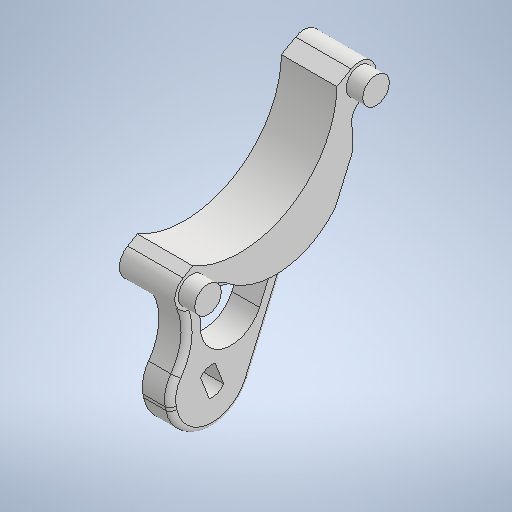
# Autodesk Inventor part: Jig
Saved by Autodesk Inventor 2025.2 (Build 292293000, 293)
## iProperties
Created: 2026-02-21
Part Number: Jig
Material: 一般
Document SubType Name: Modeling
Designer: naka6
Density: 1 g/cm^3
Appearance: 既定
Author: naka6
Autodesk Inventor part; units mm, degrees
ref_plane "YZ Plane" through (0, 0, 0) normal (1, 0, 0) x (0, 1, 0)
ref_plane "XZ Plane" through (0, 0, 0) normal (0, 1, 0) x (-1, 0, 0)
ref_plane "XY Plane" through (0, 0, 0) normal (0, 0, 1) x (1, 0, 0)
sketch "スケッチ1" plane through (0, 0, 0) normal (1, 0, 0) x (0, 1, 0)
  circle A0 centre (0, 0) radius 7.5
  circle A1 centre (0, 0) radius 2.6
  line L0 (0, 0) -> (40, 0)
  line L1 (21.0937, 8.7466) -> (38.5937, -21.5643)
  circle A2 centre (40, 0) radius 17.5
  circle A3 centre (21.0937, 8.7466) radius 3
  circle A4 centre (38.5937, -21.5643) radius 3
  line L2 (23.6918, 10.2466) -> (41.1918, -20.0643)
  line L3 (20.5133, 11.6899) -> (-1.4511, 7.3583)
  line L4 (37.4046, -24.3185) -> (-2.9729, -6.8856)
  line L5 (40, 0) -> (29.6077, -6)
  circle A5 centre (9.5821, 14.4722) radius 9.8569
  point P0 (39.7099, -17.4976)
  point P1 (24.7016, 8.4976)
  point P2 (33.2577, -13.3993)
  point P3 (37.2586, -14.7474)
  point P4 (18.9414, 11.3799)
  point P5 (2.0976, 8.0581)
  point P6 (18.4076, 10.0826)
  dimension "d0" = 15
  dimension "d1" = 5.2
  dimension "d2" = 40
  dimension "d3" = 35
  dimension "d5" = 35
  dimension "d6" = 6
  dimension "d7" = 6
  dimension "d14" = 120
  dimension "d15" = 12
  constraints: 12 end point, 8 tangent, 6 centre point, 6 point on circle, 5 coincident, 3 point on line, 1 horizontal, 1 perpendicular
  measures "d0" diameter of A0
  measures "d1" diameter of A1
  measures "d2" distance of L0.start L0.end
  measures "d3" distance of L1.start L1.end
  measures "d5" diameter of A2
  measures "d6" diameter of A3
  measures "d7" diameter of A4
  measures "d14" angle of L1 L0
  measures "d15" distance of L5.start L5.end
extrude "押し出し1" add sketch "スケッチ1" along normal blind 5 contours A0 | L3 A5 A0 | A0 L0 A2 L1 A4 L4 | A5 A3 L1 A2 L0 A0 | A4 | A3 | L1 A2 L2 A4 | A3 L2 A2 L1
sketch "スケッチ2" plane through (5, 0, 0) normal (1, 0, 0) x (0, 0, -1)
  arc A0 (24.3185, 37.4046) -> (20.0643, 41.1918) centre (21.5643, 38.5937) ccw projected
  line L0 (20.0643, 41.1918) -> (17.4976, 39.7099) projected
  arc A1 (-8.4976, 24.7016) -> (17.4976, 39.7099) centre (0, 40) ccw projected
  arc A2 (-10.2466, 23.6918) -> (-10.0826, 18.4076) centre (-8.7466, 21.0937) ccw projected
  line L1 (-8.0581, 2.0976) -> (-7.3583, -1.4511) projected
  arc A3 (-7.3583, -1.4511) -> (6.8856, -2.9729) centre (0, 0) ccw projected
  line L2 (6.8856, -2.9729) -> (24.3185, 37.4046) projected
  circle A4 centre (0, 0) radius 2.6 projected
  circle A5 centre (-8.7466, 21.0937) radius 3
  circle A6 centre (21.5643, 38.5937) radius 3
  line L3 (-8.4976, 24.7016) -> (-10.2466, 23.6918) projected
  arc A7 (-8.0581, 2.0976) -> (-10.0826, 18.4076) centre (-14.4722, 9.5821) ccw projected
  circle A8 centre (6.4088, 29.8437) radius 14
  circle A9 centre (-4.5271, 16.8281) radius 3
  circle A10 centre (23.1486, 32.8067) radius 3
  point P0 (-10.0826, 18.4076)
  point P1 (-6.6369, 18.9609)
  point P2 (-2.5972, 19.125)
  point P3 (17.207, 20.9331)
  point P4 (20.2992, 28.0951)
  point P5 (20.1945, 32.2838)
  point P6 (22.3564, 35.7002)
  dimension "d10" = 6
  dimension "d11" = 6
  dimension "d16" = 6
  dimension "d17" = 6
  dimension "d22" = 3
  dimension "d23" = 17.5
  dimension "d24" = 28
  constraints: 5 centre point, 4 tangent, 2 coincident
  measures "d10" diameter of A5
  measures "d11" diameter of A6
  measures "d16" diameter of A9
  measures "d17" diameter of A10
  measures "d22" distance from line of L0 A8.centre
  measures "d23" distance of A6.centre A8.centre
  measures "d24" diameter of A8
extrude "押し出し2" add sketch "スケッチ2" along normal blind 5 contours A6 A0 | A10 A8 A1 L0 A6 | A8 L2 A1 | A8 A9 A5 L3 A1 | A5 A2
sketch "スケッチ3" plane through (10, 0, 0) normal (1, 0, 0) x (0, 0, -1)
  arc A0 (22.3564, 35.7002) -> (20.0643, 41.1918) centre (21.5643, 38.5937) ccw projected
  circle A1 centre (21.5643, 38.5937) radius 2.4
  arc A2 (-10.2466, 23.6918) -> (-6.6369, 18.9609) centre (-8.7466, 21.0937) ccw projected
  circle A3 centre (-8.7466, 21.0937) radius 2.4
  point P0 (0, 0)
  dimension "d18" = 4.8
  dimension "d19" = 4.8
  constraints: 2 centre point, 2 coincident
  measures "d18" diameter of A1
  measures "d19" diameter of A3
extrude "押し出し3" add sketch "スケッチ3" along normal blind 3
sketch "スケッチ4" plane through (5, 0, 0) normal (1, 0, 0) x (0, 0, -1)
  circle A0 centre (0, 0) radius 2.6 projected
  line L0 (2.1005, -1.5322) -> (0.508, 2.5499)
  line L1 (-0.508, -2.5499) -> (-2.1005, 1.5322)
  line L2 (0.4478, 2.154) -> (1.7881, -1.2817) projected
  arc A1 (-0.4478, -2.154) -> (1.7881, -1.2817) centre (0, 0) ccw projected
  line L3 (-0.4478, -2.154) -> (-1.7881, 1.2817) projected
  arc A2 (0.4478, 2.154) -> (-1.7881, 1.2817) centre (0, 0) ccw projected
  dimension "d27" = 0.2
  dimension "d28" = 0.2
  constraints: 4 end point, 4 point on circle
  measures "d27" distance between parallel lines of L2 L0
  measures "d28" distance between parallel lines of L1 L3
extrude "押し出し4" add sketch "スケッチ4" against normal up to surface (5 mm away) contours A0 L0 | L1 A0
fillet "フィレット1" radius 6 1 edges at (2.5, 2.0976, 8.0581)
sketch "スケッチ5" plane through (5, 0, 0) normal (1, 0, 0) x (0, 0, -1)
  arc A0 (0.508, 2.5499) -> (-2.1005, 1.5322) centre (0, 0) ccw projected
  line L0 (0.508, 2.5499) -> (2.1005, -1.5322) projected
  arc A1 (-0.508, -2.5499) -> (2.1005, -1.5322) centre (0, 0) ccw projected
  line L1 (-0.508, -2.5499) -> (-2.1005, 1.5322) projected
  arc A2 (-6.4669, 3.8311) -> (-7.4807, -0.8305) centre (-1.5941, 0.3304) ccw projected
  line L2 (-7.4807, -0.8305) -> (-7.3583, -1.4511) projected
  arc A3 (-7.3583, -1.4511) -> (6.8856, -2.9729) centre (0, 0) ccw projected
  line L3 (6.8856, -2.9729) -> (17.207, 20.9331) projected
  arc A4 (-2.5972, 19.125) -> (17.207, 20.9331) centre (6.4088, 29.8437) ccw projected
  arc A5 (-2.5972, 19.125) -> (-6.6369, 18.9609) centre (-4.5271, 16.8281) ccw projected
  arc A6 (-10.0826, 18.4076) -> (-6.6369, 18.9609) centre (-8.7466, 21.0937) ccw projected
  arc A7 (-6.4669, 3.8311) -> (-10.0826, 18.4076) centre (-14.4722, 9.5821) ccw projected
  arc A8 (20.2992, 28.0951) -> (20.1945, 32.2838) centre (6.4088, 29.8437) ccw projected
  line L4 (20.2992, 28.0951) -> (24.3185, 37.4046) projected
  arc A9 (22.3564, 35.7002) -> (24.3185, 37.4046) centre (21.5643, 38.5937) ccw projected
  arc A10 (22.3564, 35.7002) -> (20.1945, 32.2838) centre (23.1486, 32.8067) ccw projected
  arc A11 (-4.2054, 17.2109) -> (-4.7866, 17.2555) centre (-4.5271, 16.8281) ccw
  arc A12 (-4.2054, 17.2109) -> (11.5638, 14.1697) centre (6.4088, 29.8437) ccw
  line L5 (11.5638, 14.1697) -> (4.5904, -1.9819)
  arc A13 (-4.9055, -0.9674) -> (4.5904, -1.9819) centre (0, 0) ccw
  line L6 (-4.9055, -0.9674) -> (-5.0279, -0.3468)
  arc A14 (-4.4366, 2.3725) -> (-5.0279, -0.3468) centre (-1.5941, 0.3304) ccw
  arc A15 (-4.4366, 2.3725) -> (-4.7866, 17.2555) centre (-14.4722, 9.5821) ccw
  circle A16 centre (3.4435, 9.3884) radius 5.5599
  circle A17 centre (-3.2484, 15.8531) radius 0.5
  circle A18 centre (10.6825, 13.3897) radius 0.5
  point P0 (-2.9643, 16.2645)
  point P1 (-3.6849, 15.6092)
  point P2 (-2.116, 9.4485)
  point P3 (8.548, 7.1845)
  point P4 (11.1415, 13.1915)
  point P5 (10.5568, 13.8736)
  dimension "d32" = 2.5
  dimension "d33" = 10
  dimension "d34" = 1
  dimension "d35" = 1
  constraints: 10 point on circle, 8 centre point, 6 tangent, 4 end point, 6 other
  measures "d32" radial gap between concentric circles of A7 A15
  measures "d33" distance of A16.centre point (0, 0)
  measures "d34" diameter of A17
  measures "d35" diameter of A18
extrude "押し出し5" cut sketch "スケッチ5" against normal through all contours A12 A16 A15 A17 | A17 | A12 A16 | A12 A18 L5 A16 | A18 picked at (3.6895, 10.3164)
fillet "フィレット2" radius 2 3 edges at (5, 19.8256, 4.6488) (5, 18.1317, 8.271) (5, 15.9017, -7.6817)
fillet "フィレット3" radius 1 9 edges at (5, 1.6054, 7.457) (5, -1.1408, 7.4195) (5, -7.4576, 0.7967) (5, 6.7895, -11.1005) (5.4696, 19.031, -16.3857) (8.5, 20.9331, -17.207) (5.8136, 17.7069, 8.8914) (5.0061, 16.4419, 7.3939) (5, 10.2177, 4.6358)
